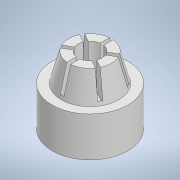
# Autodesk Inventor part: Цанга_держатель
Saved by Autodesk Inventor 2021 (Build 250183000, 183)
## iProperties
Created: 2024-03-30
Part Number: Цанга_держатель
Material: Типовые
Document SubType Name: Modeling
Designer: Мария
Density: 1 g/cm^3
Appearance: По умолчанию
Author: Мария
Autodesk Inventor part; units mm, degrees
ref_plane "YZ Plane" through (0, 0, 0) normal (1, 0, 0) x (0, 1, 0)
ref_plane "XZ Plane" through (0, 0, 0) normal (0, 1, 0) x (-1, 0, 0)
ref_plane "XY Plane" through (0, 0, 0) normal (0, 0, 1) x (1, 0, 0)
sketch "Эскиз1" plane through (0, 0, 0) normal (0, 0, 1) x (1, 0, 0)
  line L0 (17, 0) -> (17, 0)
  line L1 (6.5, 12) -> (6.5, 19.4)
  line L2 (6.5, 19.4) -> (20.4, 19.4)
  line L3 (20.4, 19.4) -> (20.4, 0)
  line L4 (0, 0) -> (0, 10)
  line L5 (17, 0) -> (17, 0)
  line L6 (6.5, 19.4) -> (6.5, 34.4)
  line L7 (6.5, 34.4) -> (11.5, 34.4)
  line L8 (11.5, 34.4) -> (15.5192, 19.4)
  line L9 (6.5, 12) -> (6.5, 0)
  line L10 (6.5, 0) -> (20.4, 0)
  point P0 (6.5, 10)
  dimension "d2" = 10
  dimension "d18" = 13
  dimension "d20" = 5
  dimension "d21" = 75
  dimension "d22" = 15
  dimension "d30" = 40.8
  dimension "d31" = 19.4
  constraints: 22 end point, 4 perpendicular, 4 vertical, 2 horizontal alignment, 1 point on line
  measures "d2" distance of L4.start L4.end
  measures "d18" diameter of L1 L4
  measures "d20" distance of L6.end L7.end
  measures "d21" angle of L8 L2
  measures "d22" distance of L1.end L6.end
  measures "d30" diameter of L3 L4
  measures "d31" distance between parallel lines of L2 L10
revolve "Вращение1" add sketch "Эскиз1" angle 360 about axis through (0, 0, 0) along (0, 1, 0)
sketch "Эскиз3" plane through (0, 34.4, 0) normal (0, 1, 0) x (1, 0, 0)
  line L0 (-1, 0) -> (1, 0)
  line L1 (1, 0) -> (1, 15)
  line L2 (1, 15) -> (-1, 15)
  line L3 (-1, 15) -> (-1, 0)
  point P0 (0, 0)
  point P1 (0, 0)
  dimension "d23" = 2
  dimension "d24" = 15
  constraints: 8 end point, 2 parallel, 1 coincident, 1 horizontal, 1 midpoint, 1 perpendicular
  measures "d23" distance between parallel lines of L1 L3
  measures "d24" distance of L0.end L1.end
extrude "Выдавливание2" cut sketch "Эскиз3" against normal up to surface (15 mm away)
pattern_circular "Круговой массив2" count 6 over 360 about axis through (0, -10, 0) along (0, 1, 0) of "Выдавливание2"
sketch "Эскиз4" plane through (0, 0, 0) normal (0, -1, 0) x (1, 0, 0)
  arc A0 (-4.3498, 16.4342) -> (-16.4073, -4.4503) centre (-0.0001, 0.0001) ccw projected
  arc A1 (16.4071, -4.45) -> (4.3493, 16.4343) centre (-0.0001, 0.0001) ccw projected
  arc A2 (2.9358, 17.8261) -> (4.3493, 16.4343) centre (4.8611, 18.3678) ccw projected
  arc A3 (2.9358, 17.8261) -> (-2.9363, 17.826) centre (-0.0003, 17.0002) ccw projected
  arc A4 (-4.3498, 16.4342) -> (-2.9363, 17.826) centre (-4.8616, 18.3676) ccw projected
  arc A5 (-16.9058, -6.3704) -> (-16.4073, -4.4503) centre (-18.3375, -4.9739) ccw projected
  arc A6 (-16.9058, -6.3704) -> (-13.9698, -11.4557) centre (-14.7225, -8.5) ccw projected
  arc A7 (-12.0576, -11.9839) -> (-13.9698, -11.4557) centre (-13.4762, -13.394) ccw projected
  arc A8 (-12.0576, -11.9839) -> (12.0576, -11.9837) centre (-0.0001, 0.0001) ccw projected
  arc A9 (13.9697, -11.4555) -> (12.0576, -11.9837) centre (13.4761, -13.3936) ccw projected
  arc A10 (13.9697, -11.4555) -> (16.9057, -6.3701) centre (14.7223, -8.4998) ccw projected
  arc A11 (16.4071, -4.45) -> (16.9057, -6.3701) centre (18.3373, -4.9736) ccw projected
extrude "Выдавливание3" cut sketch "Эскиз4" against normal blind 10.4
sketch "Эскиз5" plane through (0, 0, 0) normal (0, -1, 0) x (1, 0, 0)
  circle A0 centre (0, 0) radius 8.5 projected
  circle A1 centre (0, 0) radius 20.4 projected
  circle A2 centre (0, 0) radius 8.9
  dimension "d34" = 17.8
  constraints: 1 centre point, 1 coincident
  measures "d34" diameter of A2
extrude "Выдавливание4" add sketch "Эскиз5" along normal blind 2 contours A1
sketch "Эскиз6" plane through (0, 0, 0) normal (0, 0, 1) x (1, 0, 0)
  arc A0 (-4.445, 6.69) -> (-3.195, 5.44) centre (-3.195, 6.69) ccw projected
  line L0 (-4.445, 6.69) -> (-4.445, 7.35) projected
  arc A1 (-3.195, 8.6) -> (-4.445, 7.35) centre (-3.195, 7.35) ccw projected
  line L1 (-0.2632, 8.6) -> (-3.195, 8.6) projected
  line L2 (3.245, 8.6) -> (-0.2432, 8.6) projected
  arc A2 (4.495, 7.35) -> (3.245, 8.6) centre (3.245, 7.35) ccw projected
  line L3 (4.495, 6.69) -> (4.495, 7.35) projected
  arc A3 (3.245, 5.44) -> (4.495, 6.69) centre (3.245, 6.69) ccw projected
  line L4 (-0.0106, 8.6) -> (-0.2632, 8.6) projected
  line L5 (-3.195, 5.44) -> (3.245, 5.44) projected
  line L6 (-0.2432, 9) -> (3.245, 9)
  arc A4 (4.895, 7.35) -> (3.245, 9) centre (3.245, 7.35) ccw
  line L7 (4.895, 7.35) -> (4.895, 6.69)
  arc A5 (3.245, 5.04) -> (4.895, 6.69) centre (3.245, 6.69) ccw
  line L8 (3.245, 5.04) -> (-3.195, 5.04)
  arc A6 (-4.845, 6.69) -> (-3.195, 5.04) centre (-3.195, 6.69) ccw
  line L9 (-4.845, 6.69) -> (-4.845, 7.35)
  arc A7 (-3.195, 9) -> (-4.845, 7.35) centre (-3.195, 7.35) ccw
  line L10 (-3.195, 9) -> (-0.2632, 9)
  line L11 (-0.2432, 9) -> (-0.2632, 9)
  point P0 (0, 0)
  dimension "d37" = 1.65
  dimension "d38" = 90
  dimension "d39" = 1.65
  dimension "d42" = 4.7582
  constraints: 12 end point, 8 point on circle, 8 tangent, 4 centre point, 3 parallel, 1 horizontal
  measures "d37" radius of A4
  measures "d38" angle of L0 L6
  measures "d39" distance from line of L3.end L6
  measures "d42" distance from line of L10.end L3
extrude "Выдавливание5" cut sketch "Эскиз6" against normal through all contours L0 A1 L1 L4 L2 A2 L3 A3 L5 A0 | L6 A4 L7 A5 L8 A6 L9 A7 L10 L11
sketch "Эскиз7" plane through (0, -2, 0) normal (0, -1, 0) x (1, 0, 0)
  arc A0 (-10.8652, -13.0746) -> (10.8651, -13.0746) centre (0, 0.0001) ccw construction
  circle A1 centre (-0.0003, 17.0002) radius 1.05 projected
  circle A2 centre (14.7223, -8.4998) radius 1.05 projected
  circle A3 centre (-14.7225, -8.5) radius 1.05 projected
  circle A4 centre (-0.0003, 17.0002) radius 0.75
  circle A5 centre (14.7223, -8.4998) radius 0.75
  circle A6 centre (-14.7225, -8.5) radius 0.75
  dimension "d57" = 1.5
  dimension "d58" = 1.5
  dimension "d59" = 1.5
  constraints: 3 centre point, 3 coincident
  measures "d57" diameter of A4
  measures "d58" diameter of A5
  measures "d59" diameter of A6
extrude "Выдавливание6" cut sketch "Эскиз7" against normal blind 16 contours A4 | A5 | A6
